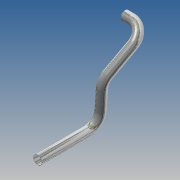
# Autodesk Inventor part: exhaust header right pipe 2
Saved by Autodesk Inventor 2013 (Build 170138000, 138)
## iProperties
Created: 2013-02-09
Part Number: exhaust header right pipe 2
Material: Steel
Document SubType Name: Modeling
Designer: zhaphod
Density: 1 g/cm^3
Author: zhaphod
Autodesk Inventor part; units mm, degrees
sketch "Sketch1" plane through (0, 0, 0) normal (1, 0, 0) x (0, 1, 0)
  line L0 (0, 0) -> (-172, -150)
  line L1 (-172, -150) -> (-172, -332.225)
  line L2 (-172, -332.225) -> (-463.85, -332.225)
  line L3 (0, 0) -> (0, -103.1875) construction
  line L4 (0, -103.1875) -> (-172, -65.475) construction
  line L5 (-172, -52.775) -> (-463.85, -52.775) construction
  dimension "d0" = 332.225
  dimension "d1" = 172
  dimension "d4" = 150
  dimension "d5" = 463.85
  dimension "d6" = 103.1875
  dimension "d7" = 52.775
  dimension "d8" = 65.475
  constraints: 12 end point, 4 vertical alignment, 2 perpendicular, 1 horizontal, 1 vertical, 2 other
  measures "d0" distance from line of L2 L0.start
  measures "d1" horizontal distance of L0.end L0.start
  measures "d4" vertical distance of L0.end L0.start
  measures "d5" horizontal distance of L0.start L2.end
  measures "d6" distance of L0.start L3.end
  measures "d7" distance from line of L5 L0.start
  measures "d8" vertical distance of L4.end L0.start
ref_plane "Work Plane1" through (103.1875, 0, 0) normal (1, 0, 0) x (0, 1, 0)
ref_plane "Work Plane2" through (65.475, 0, 0) normal (1, 0, 0) x (0, 1, 0)
ref_plane "Work Plane3" through (52.775, 0, 0) normal (1, 0, 0) x (0, 1, 0)
sketch "Sketch2" plane through (103.1875, 0, 0) normal (1, 0, 0) x (0, 1, 0)
  point P0 (0, 0)
  point P1 (0, 0)
sketch "Sketch3" plane through (65.475, 0, 0) normal (1, 0, 0) x (0, 1, 0)
  point P0 (0, 0)
  point P1 (-172, -150)
  point P2 (-172, -332.225)
sketch "Sketch4" plane through (52.775, 0, 0) normal (1, 0, 0) x (0, 1, 0)
  point P0 (0, 0)
  point P1 (-463.85, -332.225)
  point P2 (-172, -332.225)
sketch "Sketch5" plane through (0, 0, 0) normal (1, 0, 0) x (0, 1, 0)
  circle A0 centre (0, 0) radius 20.6375
  circle A1 centre (0, 0) radius 19.0375
  dimension "d15" = 1.6
  dimension "d17" = 41.275
  constraints: 2 centre point, 2 coincident
  measures "d15" radial gap between concentric circles of A0 A1
  measures "d17" diameter of A0
sketch3d "3D Sketch1"
  line L0 (0, 0, 0) -> (30.2045, 0, 0)
  arc A0 (30.2045, 0, 0) -> (91.2887, -54.2685, -47.3272) centre (30.2045, -46.6611, -40.6928) ccw
  line L1 (91.2887, -54.2685, -47.3272) -> (70.0575, -151.1, -131.7733)
  arc A1 (70.0575, -151.1, -131.7733) -> (63.5208, -172, -178.0393) centre (73.1654, -110.847, -178.7115) ccw
  line L2 (63.5208, -172, -178.0393) -> (57.0795, -172, -270.4623)
  arc A2 (57.0795, -172, -270.4623) -> (52.775, -233.9125, -332.225) centre (57.0795, -233.9125, -270.4623) ccw
  line L3 (52.775, -233.9125, -332.225) -> (52.775, -463.85, -332.225)
  dimension "d12" = 61.9125
  dimension "d13" = 61.9125
  dimension "d14" = 61.9125
sweep "Sweep1" add profiles "Sketch5" path "3D Sketch1"
equation "\"d13\" = d12"
equation "\"d14\" = d12"
equation "\"d9\" = d6"
equation "\"d10\" = d8"
equation "\"d11\" = d7"
body "Solid1"
